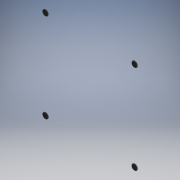
# Autodesk Inventor part: RubberFeet
Saved by Autodesk Inventor 2018 (Build 220112000, 112)
## iProperties
Created: 2019-05-03
Part Number: RubberFeet
Material: Rubber
Document SubType Name: Modeling
Designer: thatg
Density: 0.93 g/cm^3
Appearance: Rubber - Black
Author: thatg
Autodesk Inventor part; units mm, degrees
ref_plane "YZ Plane" through (0, 0, 0) normal (1, 0, 0) x (0, 1, 0)
ref_plane "XZ Plane" through (0, 0, 0) normal (0, 1, 0) x (-1, 0, 0)
ref_plane "XY Plane" through (0, 0, 0) normal (0, 0, 1) x (1, 0, 0)
sketch "Sketch1" plane through (0, 0, 0) normal (0, 0, 1) x (1, 0, 0)
  circle A0 centre (49.53, 49.53) radius 3.175 projected
  circle A1 centre (49.53, -49.53) radius 3.175 projected
  circle A2 centre (-49.53, -49.53) radius 3.175 projected
  circle A3 centre (-49.53, 49.53) radius 3.175 projected
  point P0 (0, 0)
extrude "Extrusion1" add sketch "Sketch1" along normal blind 0.254
sketch "Sketch2" plane through (-49.53, 49.53, 0.254) normal (0, 0, 1) x (1, 0, 0)
  circle A0 centre (0, 0) radius 3.175 projected
  circle A1 centre (99.06, 0) radius 3.175 projected
  circle A2 centre (99.06, -99.06) radius 3.175 projected
  circle A3 centre (0, -99.06) radius 3.175 projected
  point P0 (49.53, -49.53)
extrude "Extrusion2" add sketch "Sketch2" along normal blind 0.254
fillet "Fillet1" radius 0.254 4 edges at (46.355, -49.53, 0.508) (46.355, 49.53, 0.508) (-52.705, 49.53, 0.508) (-52.705, -49.53, 0.508)
body "Solid1"
